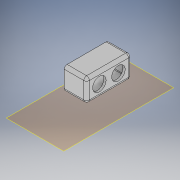
# Autodesk Inventor part: Ultrasonic Case
Saved by Autodesk Inventor 2019 (Build 230136000, 136)
## iProperties
Created: 2019-02-07
Part Number: Ultrasonic Case
Material: Generic
Document SubType Name: Modeling
Designer: Socce
Density: 1 g/cm^3
Appearance: Default
Author: Socce
Autodesk Inventor part; units mm, degrees
ref_plane "YZ Plane" through (0, 0, 0) normal (1, 0, 0) x (0, 1, 0)
ref_plane "XY Plane" through (0, 0, 0) normal (0, 0, 1) x (1, 0, 0)
ref_plane "Work Plane1" through (0, 127, 0) normal (0, 1, 0) x (-1, 0, 0)
sketch "Sketch1" plane through (0, 127, 0) normal (0, 1, 0) x (-1, 0, 0)
  line L0 (0, 0) -> (25.4, 0)
  line L1 (25.4, 0) -> (25.4, -50.8)
  line L2 (25.4, -50.8) -> (0, -50.8)
  line L3 (0, -50.8) -> (0, 0)
  dimension "d1" = 25.4
  dimension "d2" = 50.8
  constraints: 8 end point, 2 parallel, 1 horizontal, 1 perpendicular
  measures "d1" distance of L1.end L2.end
  measures "d2" distance of L0.end L1.end
extrude "Extrusion1" add sketch "Sketch1" along normal blind 25.4
fillet "Fillet1" radius 3.175 8 edges at (-12.7, 152.4, 0) (0, 139.7, 0) (0, 152.4, -25.4) (0, 139.7, -50.8) (-12.7, 152.4, -50.8) (0, 127, -25.4) (-12.7, 127, 0) (-12.7, 127, -50.8)
shell "Shell1" thickness 2.54 removed faces 0
sketch "Sketch2" plane through (0, 130.175, -47.625) normal (1, 0, 0) x (0, 0, -1)
  point P0 (-47.625, -130.175)
  point P1 (-33.1289, 9.839)
  point P2 (-11.4516, 9.7569)
hole "Hole1" at (0, 139.9319, -36.1734) at (0, 140.014, -14.4961) direction (-1, 0, 0) diameter 15.24 depth 2.54
body "Solid1"
